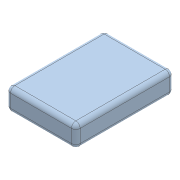
# Autodesk Inventor part: BatteryBoxSmaller
Saved by Autodesk Inventor 2018 (Build 220112000, 112)
## iProperties
Created: 2018-10-10
Part Number: BatteryBoxSmaller
Material: Generic
Document SubType Name: Modeling
Designer: Vulnic
Density: 1 g/cm^3
Appearance: Default
Author: Vulnic
Autodesk Inventor part; units mm, degrees
ref_plane "YZ Plane" through (0, 0, 0) normal (1, 0, 0) x (0, 1, 0)
ref_plane "XZ Plane" through (0, 0, 0) normal (0, 1, 0) x (-1, 0, 0)
ref_plane "XY Plane" through (0, 0, 0) normal (0, 0, 1) x (1, 0, 0)
sketch "Sketch1" plane through (0, 0, 0) normal (0, 0, 1) x (1, 0, 0)
  line L0 (-16, -22.5) -> (16, -22.5)
  line L1 (16, -22.5) -> (16, 22.5)
  line L2 (16, 22.5) -> (-16, 22.5)
  line L3 (-16, 22.5) -> (-16, -22.5)
  line L4 (-16, -22.5) -> (16, 22.5) construction
  line L5 (16, -22.5) -> (-16, 22.5) construction
  point P0 (0, 0)
  dimension "d0" = 32
  dimension "d1" = 45
  constraints: 12 end point, 2 midpoint, 2 parallel, 1 horizontal, 1 perpendicular
  measures "d0" distance between parallel lines of L1 L3
  measures "d1" distance between parallel lines of L0 L2
extrude "Extrusion1" add sketch "Sketch1" along normal blind 10
fillet "Fillet1" radius 2 12 edges at (16, 0, 10) (16, 22.5, 5) (0, 22.5, 10) (16, 0, 0) (0, 22.5, 0) (-16, 0, 0) (-16, 22.5, 5) (-16, 0, 10) (0, -22.5, 0) (0, -22.5, 10) (16, -22.5, 5) (-16, -22.5, 5)
body "Solid1"
